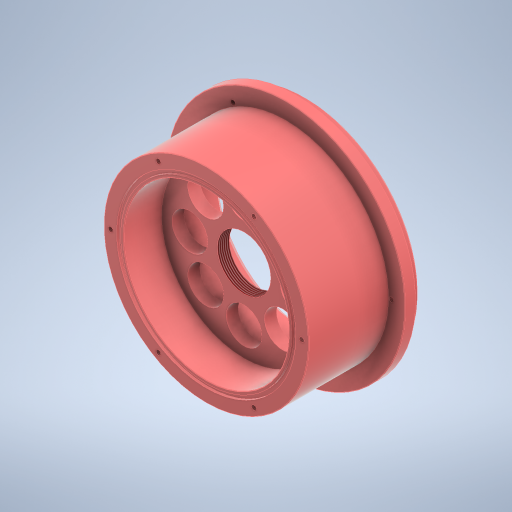
# Autodesk Inventor part: 021
Saved by Autodesk Inventor 2023 (Build 270158000, 158)
## iProperties
Created: 2021-11-06
Part Number: 021
Material: Stainless Steel, 440C
Document SubType Name: Modeling
Designer: vinicius.miguel
Density: 7.75 g/cm^3
Appearance: Smooth - Red
Mass: 1439.11 g
Surface Area: 485.602 cm^2
Volume: 185.691 cm^3
Author: vinicius.miguel
Autodesk Inventor part; units mm, degrees
ref_plane "XZ Plane" through (0, 0, 0) normal (0, 1, 0) x (-1, 0, 0)
ref_plane "XY Plane" through (0, 0, 0) normal (0, 0, 1) x (1, 0, 0)
sketch "Sketch1" plane through (0, 0, 0) normal (1, 0, 0) x (0, 1, 0)
  line L0 (0, 0) -> (0, 16.4674) construction
  line L1 (-57, -4.6) -> (-57, 0)
  line L2 (-57, 0) -> (-60, 0)
  line L3 (-60, 0) -> (-60, 5.4)
  line L4 (-60, 5.4) -> (-44.45, 5.4)
  line L5 (-44.45, 5.4) -> (-44.45, 2)
  line L6 (-44.45, 2) -> (-41.5, 2)
  line L7 (-41.5, -4.6) -> (-57, -4.6)
  line L8 (-41.5, -4.6) -> (-41.5, 2)
  line L9 (-51.5, 5.4) -> (-51.5, 45.4)
  line L10 (-51.5, 45.4) -> (-41.5, 45.4)
  line L11 (-41.5, 45.4) -> (-41.5, 2)
  line L12 (-45, 45.4) -> (-45, 44.2)
  line L13 (-45, 44.2) -> (-43, 44.2)
  line L14 (-43, 44.2) -> (-43, 45.4)
  line L15 (-41.5, 26.4) -> (-13, 26.4)
  line L16 (-13, 26.4) -> (-13, 20.4)
  line L17 (-13, 20.4) -> (-41.5, 20.4)
  point P0 (-47.5615, 5.4)
  dimension "d2" = 4.6
  dimension "d3" = 10
  dimension "d8" = 88.9
  dimension "d9" = 120
  dimension "d20" = 114
  dimension "d40" = 2
  dimension "d44" = 83
  dimension "d45" = 50
  dimension "d46" = 10
  dimension "d68" = 86
  dimension "d69" = 2
  dimension "d70" = 1.2
  dimension "d81" = 6
  dimension "d82" = 25
  dimension "d83" = 26
  constraints: 36 end point, 12 perpendicular, 5 point on line, 4 vertical, 1 horizontal, 1 horizontal alignment
  measures "d2" distance of L1.start L1.end
  measures "d3" distance between parallel lines of L4 L7
  measures "d8" diameter of L5 L0
  measures "d9" diameter of L3 L0
  measures "d20" diameter of L1 L0
  measures "d40" distance between parallel lines of L2 L6
  measures "d44" diameter of L11 L0
  measures "d45" distance between parallel lines of L7 L10
  measures "d46" distance of L9.end L10.end
  measures "d68" diameter of L14 L0
  measures "d69" distance of L12.end L13.end
  measures "d70" distance of L13.end L14.end
  measures "d81" distance of L15.end L16.end
  measures "d82" distance between parallel lines of L17 L7
  measures "d83" diameter of L16 L0
revolve "Revolution1" add sketch "Sketch1" angle 360 about axis through (0, 0, 0) along (0, 0, 1)
chamfer "Chamfer4" distance 1 angle 45 1 edges at (0, 57, -4.6)
sketch "Sketch2" plane through (0, 0, -4.6) normal (0, 0, -1) x (-1, 0, 0)
  point P0 (0, 0)
  point P1 (-53, 0)
  dimension "d26" = 53
  constraints: 1 horizontal alignment
  measures "d26" distance of point (0, 0) point (-53, 0)
hole "Hole1" at (53, 0, -4.6) direction (0, 0, 1) diameter 2.459 end through all counterbore diameter 4 counterbore depth 4.6 thread size "M3x0.5" class "6H" standard "ANSI Metric M Profile"
pattern_circular "Circular Pattern1" count 3 over 360 about axis through (0, 0, 2.7) along (0, 0, 1) of "Hole1"
chamfer "Chamfer5" distance 3 angle 45 1 edges at (0, 41.5, -4.6)
sketch "Sketch3" plane through (0, 0, 45.4) normal (0, 0, 1) x (1, 0, 0)
  circle A0 centre (0, 0) radius 51.5 projected
  circle A1 centre (0, 0) radius 41.5 projected
  circle A2 centre (0, 0) radius 51.5 projected
  point P0 (48, 0)
  dimension "d65" = 48
  constraints: 1 horizontal alignment
  measures "d65" distance of point (48, 0) point (0, 0)
hole "Hole2" at (48, 0, 45.4) direction (0, 0, -1) diameter 2.459 depth 8.8 tip angle 118 thread size "M3x0.5" class "6H" standard "ISO Metric profile"
pattern_circular "Circular Pattern2" count 6 over 360 about axis through (0, 0, 25.4) along (0, 0, 1) of "Hole2"
ref_plane "Work Plane1" through (-51.5, 0, 25.4) normal (1, 0, 0) x (0, 1, 0)
chamfer "Chamfer6" distance 0.25 angle 45 4 edges at (0, 51.5, 45.4) (0, 41.5, 45.4) (0, 60, 5.4) (0, 60, 0)
sketch "Sketch7" plane through (0, 0, 20.4) normal (0, 0, -1) x (-1, 0, 0)
  circle A0 centre (27.25, 0) radius 9
  circle A1 centre (0, 0) radius 41.5 projected
  circle A2 centre (0, 0) radius 13 projected
  circle A3 centre (0, 0) radius 41.5 projected
  line L0 (41.5, 0) -> (13, 0) construction
  dimension "d84" = 18
  constraints: 3 horizontal alignment, 2 end point, 1 centre point, 1 coincident, 1 horizontal, 1 midpoint, 2 other
  measures "d84" diameter of A0
extrude "Extrusion3" cut sketch "Sketch7" against normal blind 10 contours A0
pattern_circular "Circular Pattern3" count 8 over 360 about axis through (0, 0, 23.4) along (0, 0, 1) of "Extrusion3"
sketch "Sketch8" plane through (0, 0, 26.4) normal (0, 0, 1) x (1, 0, 0)
  circle A0 centre (0, 0) radius 13 projected
  constraints: 1 coincident
hole "Hole4" at (0, 0, 26.4) direction (0, 0, -1) diameter 26.9175 end through all thread size "M28x1" class "6H" standard "ISO Metric profile"
sketch "Sketch9" plane through (0, 0, 45.4) normal (0, 0, 1) x (1, 0, 0)
  circle A0 centre (0, 0) radius 43
  circle A1 centre (0, 0) radius 45
  dimension "d97" = 86
  dimension "d98" = 2
  constraints: 2 centre point, 1 coincident
  measures "d97" diameter of A0
  measures "d98" radial gap between concentric circles of A0 A1
extrude "Extrusion4" cut sketch "Sketch9" against normal blind 1.23
body "Solid1"
